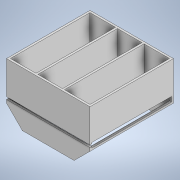
# Autodesk Inventor part: BeadCompartments_4
Saved by Autodesk Inventor 2020 (Build 240168000, 168)
## iProperties
Created: 2022-01-22
Part Number: BeadCompartments_4
Material: Generic
Document SubType Name: Modeling
Designer: danie
Density: 1 g/cm^3
Appearance: Default
Author: danie
Autodesk Inventor part; units mm, degrees
ref_plane "YZ Plane" through (0, 0, 0) normal (1, 0, 0) x (0, 1, 0)
ref_plane "XZ Plane" through (0, 0, 0) normal (0, 1, 0) x (-1, 0, 0)
ref_plane "XY Plane" through (0, 0, 0) normal (0, 0, 1) x (1, 0, 0)
sketch "Sketch2" plane through (0, 0, 0) normal (0, 1, 0) x (-1, 0, 0)
  line L0 (0, 0) -> (-127, 0)
  line L1 (-127, 0) -> (-127, -127)
  line L2 (-127, -127) -> (0, -127)
  line L3 (0, -127) -> (0, 0)
  line L4 (0, 0) -> (-40.7416, 0)
  line L5 (-40.7416, 0) -> (-40.7416, -127)
  line L6 (-40.7416, -127) -> (0, -127)
  line L7 (0, -127) -> (0, 0)
  line L8 (3.175, 3.175) -> (-130.175, 3.175)
  line L9 (-130.175, 3.175) -> (-130.175, -130.175)
  line L10 (-130.175, -130.175) -> (3.175, -130.175)
  line L11 (3.175, -130.175) -> (3.175, 3.175)
  line L12 (-127, 0) -> (-86.2584, 0)
  line L13 (-86.2584, 0) -> (-86.2584, -127)
  line L14 (-86.2584, -127) -> (-127, -127)
  line L15 (-127, -127) -> (-127, 0)
  line L16 (-40.7416, -44.9087) -> (-43.9166, -44.9087) construction
  line L17 (-86.2584, -51.4533) -> (-83.0834, -51.4533) construction
  line L18 (-43.9166, 0) -> (-83.0834, 0)
  line L19 (-83.0834, 0) -> (-83.0834, -127)
  line L20 (-83.0834, -127) -> (-43.9166, -127)
  line L21 (-43.9166, -127) -> (-43.9166, 0)
  dimension "d11" = 127
  dimension "d12" = 127
  dimension "d13" = 40.7416
  dimension "d14" = 3.175
  dimension "d15" = 40.7416
  dimension "d16" = 3.175
  dimension "d17" = 3.175
  constraints: 44 end point, 10 parallel, 7 perpendicular, 6 point on line, 4 horizontal, 3 other
  measures "d11" distance of L2.end L1.end
  measures "d12" distance of L1.end L0.end
  measures "d13" distance of L6.end L5.end
  measures "d14" distance between parallel lines of L3 L11
  measures "d15" distance of L13.end L14.end
  measures "d16" distance of L16.start L16.end
  measures "d17" distance of L17.start L17.end
extrude "Extrusion2" add sketch "Sketch2" along normal blind 50.8 contours L5 L2 L21 L0 | L19 L2 L13 L0 | L11 L10 L9 L8
sketch "Sketch3" plane through (0, 0, 0) normal (0, -1, 0) x (1, 0, 0)
  line L0 (130.175, 3.175) -> (130.175, -130.175) projected
  line L1 (-3.175, -130.175) -> (-3.175, 3.175) projected
  line L2 (130.175, 3.175) -> (-3.175, 3.175)
  line L3 (-3.175, 3.175) -> (-3.175, 0)
  line L4 (-3.175, 0) -> (130.175, 0)
  line L5 (130.175, 0) -> (130.175, 3.175)
  line L6 (130.175, -130.175) -> (-3.175, -130.175)
  line L7 (-3.175, -130.175) -> (-3.175, -127)
  line L8 (-3.175, -127) -> (130.175, -127)
  line L9 (130.175, -127) -> (130.175, -130.175)
  point P0 (0, 0)
  dimension "d20" = 133.35
  dimension "d21" = 3.175
  constraints: 16 end point, 4 parallel, 2 horizontal, 2 perpendicular, 1 point on line
  measures "d20" distance of L7.end L8.end
  measures "d21" distance of L6.end L7.end
extrude "Extrusion3" add sketch "Sketch3" along normal blind 1.905 contours L0 L4 L1 L2
sketch "Sketch4" plane through (0, 0, 0) normal (0, -1, 0) x (1, 0, 0)
  line L0 (130.175, 0) -> (130.175, -130.175) projected
  line L1 (130.175, -130.175) -> (-3.175, -130.175)
  line L2 (-3.175, -130.175) -> (-3.175, -127)
  line L3 (-3.175, -127) -> (130.175, -127)
  line L4 (130.175, -127) -> (130.175, -130.175)
  point P0 (0, 0)
  dimension "d24" = 133.35
  dimension "d25" = 3.175
  constraints: 8 end point, 2 parallel, 1 horizontal, 1 perpendicular
  measures "d24" distance of L2.end L3.end
  measures "d25" distance of L1.end L2.end
extrude "Extrusion4" add sketch "Sketch4" along normal blind 7.62
sketch "Sketch5" plane through (0, -7.62, 0) normal (0, -1, 0) x (1, 0, 0)
  line L0 (130.175, -130.175) -> (-3.175, -130.175) projected
  line L1 (130.175, -130.175) -> (-3.175, -130.175)
  line L2 (-3.175, -130.175) -> (-3.175, 3.175)
  line L3 (-3.175, 3.175) -> (130.175, 3.175)
  line L4 (130.175, 3.175) -> (130.175, -130.175)
  line L5 (127, 0) -> (0, 0)
  line L6 (0, 0) -> (0, -127)
  line L7 (0, -127) -> (127, -127)
  line L8 (127, -127) -> (127, 0)
  point P0 (0, 0)
  dimension "d32" = 3.175
  constraints: 16 end point, 4 parallel, 2 perpendicular, 1 horizontal, 3 other
  measures "d32" distance between parallel lines of L3 L5
extrude "Extrusion5" add sketch "Sketch5" along normal blind 3.175
sketch "Sketch6" plane through (0, -10.795, 0) normal (0, -1, 0) x (1, 0, 0)
  line L0 (130.175, -127) -> (130.175, 3.175) projected
  line L1 (-3.175, -130.175) -> (-3.175, 3.175) projected
  line L2 (130.175, 3.175) -> (-3.175, 3.175)
  line L3 (-3.175, 3.175) -> (-3.175, 0)
  line L4 (-3.175, 0) -> (130.175, 0)
  line L5 (130.175, 0) -> (130.175, 3.175)
  point P0 (0, 0)
  constraints: 8 end point, 2 parallel, 1 horizontal, 1 perpendicular, 1 point on line
extrude "Extrusion6" add sketch "Sketch6" against normal blind 5.08
sketch "Sketch7" plane through (-3.175, -10.795, 3.175) normal (0, 0, 1) x (1, 0, 0)
  line L0 (0, 0) -> (133.35, 0) construction
  line L1 (0, 0) -> (0, -25.4) construction
  line L2 (0, -25.4) -> (25.4, -25.4) construction
  line L3 (133.35, 0) -> (133.35, -25.4) construction
  line L4 (133.35, -25.4) -> (107.95, -25.4) construction
  line L5 (0, 0) -> (25.4, -25.4)
  line L6 (25.4, -25.4) -> (107.95, -25.4)
  line L7 (107.95, -25.4) -> (133.35, 0)
  line L8 (0, 0) -> (133.35, 0)
  point P0 (3.175, 10.795)
  dimension "d33" = 25.4
  dimension "d34" = 25.4
  dimension "d35" = 25.4
  dimension "d36" = 25.4
  constraints: 16 end point, 2 vertical, 1 horizontal, 1 perpendicular
  measures "d33" distance of L0.start L1.end
  measures "d34" distance of L1.end L2.end
  measures "d35" distance of L0.end L3.end
  measures "d36" distance of L3.end L4.end
extrude "Extrusion7" add sketch "Sketch7" against normal blind 3.175
sketch "Sketch8" plane through (130.175, 50.8, -130.175) normal (0, 0, -1) x (-1, 0, 0)
  line L0 (107.95, -86.995) -> (133.35, -61.595) projected
  line L1 (133.35, -61.595) -> (107.95, -86.995)
  line L2 (25.4, -86.995) -> (107.95, -86.995) projected
  line L3 (107.95, -86.995) -> (25.4, -86.995)
  line L4 (0, -56.515) -> (0, -61.595) projected
  line L5 (25.4, -86.995) -> (0, -61.595)
  line L6 (0, -61.595) -> (133.35, -61.595)
  point P0 (130.175, -50.8)
  constraints: 8 end point, 2 collinear, 2 perpendicular
extrude "Extrusion8" add sketch "Sketch8" against normal blind 3.175
sketch "Sketch9" plane through (22.225, -36.195, -127) normal (-0.7071068, -0.7071068, 0) x (-0.7071068, 0.7071068, 0)
  line L0 (35.921, 0) -> (35.921, 3.175) projected
  line L1 (39.5131, -130.175) -> (-54.7796, -130.175) projected
  line L2 (35.921, 3.175) -> (-0.0076, 3.175)
  line L3 (-0.0076, 3.175) -> (-0.0076, -130.175)
  line L4 (-0.0076, -130.175) -> (35.921, -130.175)
  line L5 (35.921, -130.175) -> (35.921, 3.175)
  point P0 (41.3092, -127)
  point P1 (35.921, -130.175)
  point P2 (35.921, 0)
  constraints: 8 end point, 2 parallel, 1 horizontal, 1 perpendicular, 1 point on line
extrude "Extrusion9" add sketch "Sketch9" against normal blind 3.175
sketch "Sketch10" plane through (104.775, -36.195, 3.175) normal (0.7071068, -0.7071068, 0) x (-0.7071068, -0.7071068, 0)
  line L0 (0, 0) -> (0, 3.175) projected
  line L1 (-35.921, 133.35) -> (0, 133.35) projected
  line L2 (0, 0) -> (-35.921, 0)
  line L3 (-35.921, 0) -> (-35.921, 133.35)
  line L4 (-35.921, 133.35) -> (0, 133.35)
  line L5 (0, 133.35) -> (0, 0)
  point P0 (48.4934, 3.175)
  constraints: 8 end point, 2 parallel, 1 horizontal, 1 perpendicular
extrude "Extrusion10" add sketch "Sketch10" against normal blind 3.175
body "Solid2"
